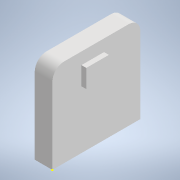
# Autodesk Inventor part: new tal lpart
Saved by Autodesk Inventor 2022 (Build 260153000, 153)
## iProperties
Created: 2023-06-20
Part Number: new tal lpart
Material: Generic
Document SubType Name: Modeling
Designer: vidya
Density: 1 g/cm^3
Appearance: Default
Author: vidya
Autodesk Inventor part; units mm, degrees
ref_plane "YZ Plane" through (0, 0, 0) normal (1, 0, 0) x (0, 1, 0)
ref_plane "XZ Plane" through (0, 0, 0) normal (0, 1, 0) x (-1, 0, 0)
ref_plane "XY Plane" through (0, 0, 0) normal (0, 0, 1) x (1, 0, 0)
sketch "Sketch1" plane through (0, 0, 0) normal (1, 0, 0) x (0, 1, 0)
  point P0 (0, 0)
sketch "Sketch2" plane through (0, 0, 0) normal (0, 1, 0) x (-1, 0, 0)
  line L0 (0, 0) -> (91.44, 0)
  line L1 (91.44, 0) -> (91.44, -457.2)
  line L2 (91.44, -457.2) -> (0, -457.2)
  line L3 (0, -457.2) -> (0, 0)
  dimension "d0" = 91.44
  dimension "d1" = 457.2
  constraints: 8 end point, 2 parallel, 1 horizontal, 1 perpendicular
  measures "d0" distance of L1.end L2.end
  measures "d1" distance of L0.end L1.end
extrude "Extrusion1" add sketch "Sketch2" along normal blind 457.2
fillet "Fillet1" radius 60.96 2 edges at (-45.72, 457.2, 0) (-45.72, 457.2, -457.2)
sketch "Sketch3" plane through (0, 0, 0) normal (1, 0, 0) x (0, 0, -1)
  line L0 (150.961, 395.9055) -> (268.4404, 395.9055)
  line L1 (268.4404, 395.9055) -> (268.4404, 300.7472)
  line L2 (268.4404, 300.7472) -> (150.961, 300.7472)
  line L3 (150.961, 300.7472) -> (150.961, 395.9055)
  point P0 (0, 0)
  constraints: 8 end point, 2 parallel, 1 horizontal, 1 perpendicular
extrude "Extrusion2" add sketch "Sketch3" along normal blind 25.4
body "Solid1"
